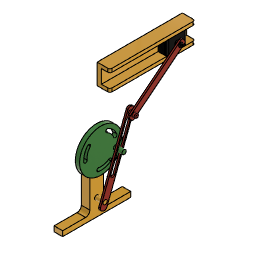
Quick return mechanism (Autodesk Fusion 360 design; units mm, degrees)
Autodesk Fusion 360 part; units mm, degrees
sketch "Sketch1" plane through (0, 0, 0) normal (1, 0, 0) x (0, 1, 0)
  circle A0 centre (0, 0) radius 25
  arc A1 (11.6807, 11.3131) -> (0, 16.2611) centre (0, 0) ccw
  arc A2 (14.3893, 14.0961) -> (0, 20.1433) centre (0, 0) ccw
  arc A3 (11.6807, 11.3131) -> (13.7011, 14.7659) centre (12.6909, 13.0395) ccw
  arc A4 (0, 20.1433) -> (0, 16.2611) centre (0, 18.2022) ccw
  arc A5 (-15.6377, 4.4592) -> (-19.6382, 4.4826) centre (-17.638, 4.4709) ccw
  arc A6 (-15.6377, 4.4592) -> (-14.0825, -8.1306) centre (0, 0) ccw
  arc A7 (-17.4446, -10.0716) -> (-14.0825, -8.1306) centre (-15.7636, -9.1011) ccw
  arc A8 (-19.4022, 5.4134) -> (-17.4446, -10.0716) centre (0, 0) ccw
  arc A9 (3.9571, -15.7723) -> (5.9371, -19.2484) centre (4.9471, -17.5104) ccw
  arc A10 (3.9571, -15.7723) -> (14.0825, -8.1306) centre (0, 0) ccw
  arc A11 (17.4446, -10.0716) -> (14.0825, -8.1306) centre (15.7636, -9.1011) ccw
  arc A12 (5.0129, -19.5095) -> (17.4446, -10.0716) centre (0, 0) ccw
  circle A13 centre (-11.0717, 14.1921) radius 2.5
  circle A14 centre (0, 0) radius 18 construction
  dimension "d1" = 50
  dimension "d3" = 360
  dimension "d4" = 5
  dimension "d6" = 36
  constraint coincident A0.centre A1.centre
  constraint concentric A0 A2
  constraint tangent A2 A4
  constraint coincident A2.start A3
  constraint coincident A2 A3.end
  constraint concentric A2 A14
  constraint coincident A13.centre A14
  measures "d1" diameter of A0
  measures "d4" diameter of A13
  measures "d6" diameter of A14
extrude "Extrude1" add sketch "Sketch1" along normal blind 5 contours A0 | A13 makes body 1
extrude "Extrude2" add sketch "Sketch1" along normal blind 15 contours A13 bodies 1
sketch "Sketch2" plane through (0, 0, 0) normal (1, 0, 0) x (0, 1, 0)
  circle A0 centre (0, 0) radius 5
  dimension "d11" = 10
  constraint coincident A0.centre origin
  measures "d11" diameter of A0
extrude "Extrude3" add sketch "Sketch2" against normal blind 10 bodies 1
sketch "Sketch1 (2)" plane through (0, 0, 0) normal (1, 0, 0) x (0, 1, 0) in component "Component"
  line L0 (-3, 10) -> (3, 10)
  line L1 (8, 5) -> (8, -59)
  line L2 (-8, -59) -> (-8, 5)
  line L3 (40, -64) -> (40, -70)
  line L4 (40, -70) -> (-40, -70)
  line L5 (-40, -70) -> (-40, -64)
  line L6 (-40, -64) -> (-13, -64)
  line L7 (13, -64) -> (40, -64)
  arc A0 (-3, 10) -> (-8, 5) centre (-3, 5) ccw
  arc A1 (8, 5) -> (3, 10) centre (3, 5) ccw
  arc A2 (-13, -64) -> (-8, -59) centre (-13, -59) ccw
  arc A3 (8, -59) -> (13, -64) centre (13, -59) ccw
  circle A4 centre (0, -50) radius 2.5
  circle A5 centre (0, 0) radius 5
  dimension "d14" = 16
  dimension "d15" = 8
  dimension "d16" = 80
  dimension "d17" = 80
  dimension "d18" = 32
  dimension "d19" = 6
  dimension "d20" = 10
  dimension "d21" = 5
  dimension "d24" = 5
  dimension "d25" = 8
  dimension "d26" = 20
  dimension "d71" = 10
  dimension "d88" = 0
  dimension "d89" = 0
  dimension "d90" = 0
  dimension "d91" = 0
  constraint horizontal L0
  constraint vertical L1
  constraint vertical L2
  constraint horizontal L6
  constraint vertical L3
  constraint horizontal L4
  constraint vertical L5
  constraint collinear L6 L7
  constraint tangent L0 A0
  constraint tangent L2 A0
  constraint tangent L0 A1
  constraint tangent L1 A1
  constraint equal A0 A1
  constraint tangent L2 A2
  constraint tangent L6 A2
  constraint equal A0 A2
  constraint tangent L1 A3
  constraint tangent L7 A3
  constraint equal A0 A3
  constraint coincident A5.centre origin
  measures "d14" distance of L1 L2
  measures "d15" distance of A5.centre L1
  measures "d16" distance of L0 L4
  measures "d17" distance of L3 L5
  measures "d18" distance of L2 L5
  measures "d19" distance of L4 L6
  measures "d20" distance of A5.centre L0
  measures "d21" radius of A0
  measures "d24" diameter of A4
  measures "d25" distance of L1 A4.centre
  measures "d26" distance of L4 A4.centre
  measures "d71" diameter of A5
extrude "Extrude1'" add sketch "Sketch1 (2)" against normal blind 10 separate body contours L0 L1 L2 L3 L4 L5 L6 L7 A0 A1 A2 A3 | A4 makes body 2 in component "Component"
extrude "Extrude2'" add sketch "Sketch1 (2)" along normal blind 10 contours A4 bodies 2 in component "Component"
sketch "Sketch1 (3)" plane through (0, 0, 0) normal (1, 0, 0) x (0, 1, 0) in component "Component'"
  circle A0 centre (0, -50) radius 2.5
  arc A1 (8, 5) -> (3, 10) centre (3, 5) ccw
  line L0 (3, 10) -> (-3, 10)
  arc A2 (-3, 10) -> (-8, 5) centre (-3, 5) ccw
  line L1 (-8, 5) -> (-8, -59)
  arc A3 (-13, -64) -> (-8, -59) centre (-13, -59) ccw
  line L2 (-13, -64) -> (-40, -64)
  line L3 (-40, -64) -> (-40, -70)
  line L4 (-40, -70) -> (40, -70)
  line L5 (40, -70) -> (40, -64)
  line L6 (40, -64) -> (13, -64)
  arc A4 (8, -59) -> (13, -64) centre (13, -59) ccw
  line L7 (8, -59) -> (8, 5)
  line L8 (-1, 38) -> (1, 38)
  line L9 (4, 35) -> (4, -55)
  line L10 (1, -58) -> (-1, -58)
  line L11 (-4, -55) -> (-4, 35)
  arc A5 (-1, 38) -> (-4, 35) centre (-1, 35) ccw
  arc A6 (4, 35) -> (1, 38) centre (1, 35) ccw
  arc A7 (-4, -55) -> (-1, -58) centre (-1, -55) ccw
  arc A8 (1, -58) -> (4, -55) centre (1, -55) ccw
  circle A9 centre (0, -50) radius 2.5
  line L12 (2.5, -24.977) -> (2.5, 25.023)
  arc A10 (2.5, 25.023) -> (-2.5, 25.023) centre (0, 25.023) ccw
  line L13 (-2.5, 25.023) -> (-2.5, -24.977)
  arc A11 (-2.5, -24.977) -> (2.5, -24.977) centre (0, -24.977) ccw
  line L14 (0, -24.977) -> (0, 25.023) construction
  circle A12 centre (0, 32) radius 2.5
  circle A13 centre (0, 0) radius 5
  dimension "d29" = 8
  dimension "d30" = 96
  dimension "d31" = 12
  dimension "d32" = 4
  dimension "d33" = 3
  dimension "d34" = 5
  dimension "d35" = 4
  dimension "d36" = 50
  dimension "d37" = 5
  dimension "d38" = 6
  dimension "d84" = 0
  dimension "d85" = 0
  dimension "d86" = 0
  dimension "d87" = 0
  constraint horizontal L8
  constraint vertical L9
  constraint horizontal L10
  constraint vertical L11
  constraint tangent L8 A5
  constraint tangent L11 A5
  constraint tangent L8 A6
  constraint tangent L9 A6
  constraint equal A5 A6
  constraint tangent L10 A7
  constraint tangent L11 A7
  constraint equal A5 A7
  constraint tangent L9 A8
  constraint tangent L10 A8
  constraint equal A5 A8
  constraint concentric A0 A9
  constraint tangent L12 A10
  constraint tangent A10 L13
  constraint parallel L12 L13
  constraint tangent L13 A11
  constraint tangent L12 A11
  constraint perpendicular L0 L14
  measures "d29" distance of L9 L11
  measures "d30" distance of L8 L10
  measures "d31" distance of L4 L10
  measures "d32" distance of L1 L11
  measures "d33" radius of A5
  measures "d34" distance of L12 L13
  measures "d35" distance of L11 A11.centre
  measures "d36" distance of A11.centre A10.centre
  measures "d37" diameter of A12
  measures "d38" distance of L8 A12.centre
extrude "Extrude1''" add sketch "Sketch1 (3)" along normal blind 2 separate body contours A1 L0 L9 L12 A13 | A1 L0 A2 L8 L9 L11 A5 A6 L12 A10 L13 | L9 L12 A13 | L9 L10 L11 A7 A8 L12 L13 A11 A13 | L0 A2 L11 L13 A13 | L11 L13 A13 makes body 3 in component "Component'"
extrude "Extrude2''" add sketch "Sketch1 (3)" along normal blind 10 contours A12 bodies 3 in component "Component'"
fillet "Fillet1" radius 1 1 edges at (10, -2.3308, 31.096) on bodies 3 in component "Component'"
sketch "Sketch1 (4)" plane through (0, 0, 0) normal (1, 0, 0) x (0, 1, 0) in component "Component''"
  line L0 (-7.9669, 51.3332) -> (68.0331, 51.3332)
  line L1 (70.0331, 49.3332) -> (70.0331, 46.3332)
  line L2 (68.0331, 44.3332) -> (-7.9669, 44.3332)
  line L3 (-9.9669, 46.3332) -> (-9.9669, 49.3332)
  circle A0 centre (-4.9669, 47.8332) radius 2.5
  circle A1 centre (65.0331, 47.8332) radius 2.5
  line L4 (-9.9669, 47.8332) -> (70.0331, 47.8332) construction
  arc A2 (-7.9669, 51.3332) -> (-9.9669, 49.3332) centre (-7.9669, 49.3332) ccw
  arc A3 (-9.9669, 46.3332) -> (-7.9669, 44.3332) centre (-7.9669, 46.3332) ccw
  arc A4 (68.0331, 44.3332) -> (70.0331, 46.3332) centre (68.0331, 46.3332) ccw
  arc A5 (70.0331, 49.3332) -> (68.0331, 51.3332) centre (68.0331, 49.3332) ccw
  dimension "d44" = 80
  dimension "d45" = 7
  dimension "d46" = 5
  dimension "d47" = 5
  dimension "d48" = 5
  dimension "d49" = 5
  dimension "d50" = 2
  constraint horizontal L0
  constraint vertical L1
  constraint horizontal L2
  constraint vertical L3
  constraint coincident A0.centre L4
  constraint coincident A1.centre L4
  constraint coincident L3 L4.start
  constraint tangent L0 A2
  constraint tangent L3 A2
  constraint tangent L2 A3
  constraint tangent L3 A3
  constraint equal A2 A3
  constraint coincident L1 L4.end
  constraint tangent L1 A4
  constraint tangent L2 A4
  constraint equal A2 A4
  constraint tangent L0 A5
  constraint tangent L1 A5
  constraint equal A2 A5
  measures "d44" distance of L1 L3
  measures "d45" distance of L0 L2
  measures "d46" diameter of A0
  measures "d47" diameter of A1
  measures "d48" distance of L3 A0.centre
  measures "d49" distance of L1 A1.centre
  measures "d50" radius of A2
extrude "Extrude1'''" add sketch "Sketch1 (4)" along normal blind 2 separate body makes body 4 in component "Component''"
sketch "Sketch1 (5)" plane through (0, 0, 0) normal (1, 0, 0) x (0, 1, 0) in component "Component'''"
  line L0 (26.7686, 78.2209) -> (126.7686, 78.2209)
  line L1 (126.7686, 78.2209) -> (126.7686, 54.2209)
  line L2 (126.7686, 54.2209) -> (26.7686, 54.2209)
  line L3 (26.7686, 54.2209) -> (26.7686, 78.2209)
  line L4 (26.7686, 74.2209) -> (126.7686, 74.2209)
  line L5 (26.7686, 58.2209) -> (126.7686, 58.2209)
  dimension "d53" = 100
  dimension "d54" = 24
  dimension "d55" = 4
  dimension "d56" = 4
  constraint horizontal L0
  constraint vertical L1
  constraint horizontal L2
  constraint vertical L3
  constraint coincident L3 L4.start
  constraint coincident L1 L4.end
  constraint perpendicular L1 L4
  constraint coincident L3 L5.start
  constraint coincident L1 L5.end
  constraint perpendicular L1 L5
  measures "d53" distance of L1 L3
  measures "d54" distance of L0 L2
  measures "d55" distance of L0 L4
  measures "d56" distance of L2 L5
extrude "Extrude1''''" add sketch "Sketch1 (5)" against normal blind 5 separate body makes body 5 in component "Component'''"
extrude "Extrude2'''" add sketch "Sketch1 (5)" along normal blind 10 contours L0 L1 L3 L4 | L1 L2 L3 L5 bodies 5 in component "Component'''"
fillet "Fillet1'" radius 2.5 4 edges at (10, 26.7686, 76.2209) (10, 26.7686, 56.2209) (10, 126.7686, 76.2209) (10, 126.7686, 56.2209) on bodies 5 in component "Component'''"
sketch "Sketch1 (6)" plane through (0, 76.7686, 66.2209) normal (1, 0, 0) x (0, 1, 0) in component "Component''''"
  line L0 (7.766, 7.3734) -> (31.766, 7.3734)
  line L1 (31.766, 7.3734) -> (31.766, -8.6266)
  line L2 (31.766, -8.6266) -> (7.766, -8.6266)
  line L3 (7.766, -8.6266) -> (7.766, 7.3734)
  circle A0 centre (19.766, -0.6266) radius 2.5
  dimension "d62" = 16
  dimension "d63" = 24
  dimension "d64" = 5
  constraint horizontal L0
  constraint vertical L1
  constraint horizontal L2
  constraint vertical L3
  measures "d62" distance of L0 L2
  measures "d63" distance of L1 L3
  measures "d64" diameter of A0
extrude "Extrude1'''''" add sketch "Sketch1 (6)" along normal blind 10 separate body contours L0 L1 L2 L3 | A0 makes body 6 in component "Component''''"
extrude "Extrude2''''" add sketch "Sketch1 (6)" along normal blind 15 contours A0 bodies 6 in component "Component''''"
fillet "Fillet1''" radius 1.5 1 edges at (15, 94.2037, 64.6903) on bodies 6 in component "Component''''"
fillet "Fillet2" radius 2.5 2 edges at (10, 84.5346, 65.5943) (10, 108.5346, 65.5943) on bodies 6 in component "Component''''"
copy_body "Body->Comp1" bodies 1 removing the originals makes body 7 in component "Component'''''"
component "Component" placed x (1, 0, 0) y (0, 1, 0) z (0, 0, 1) at (0, 0, 0)
component "Component'" placed x (1, 0, 0) y (0, 0.990399, -0.138239) z (0, 0.138239, 0.990399) at (8, 6.9119, -0.4801)
component "Component''" placed x (1, 0, 0) y (0, 0.830944, 0.556357) z (0, -0.556357, 0.830944) at (12.5, 42.0751, -5.7707)
component "Component'''" placed x (1, 0, 0) y (0, 1, 0) z (0, 0, 1) at (0, -21.198, 3.9368)
component "Component''''" placed x (1, 0, 0) y (0, 1, 0) z (0, 0, 1) at (0, -27.0329, 4.5633)
component "Component'''''" placed x (1, 0, 0) y (0, 0.366724, -0.93033) z (0, 0.93033, 0.366724) at (0, 0, 0)
